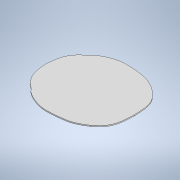
# Autodesk Inventor part: head_1
Saved by Autodesk Inventor 2020 (Build 240168000, 168)
## iProperties
Created: 2022-02-10
Part Number: head_1
Material: Типовые
Document SubType Name: Modeling
Designer: HP
Density: 1 g/cm^3
Appearance: По умолчанию
Mass: 318.083 g
Surface Area: 1630.63 cm^2
Volume: 318.083 cm^3
Author: HP
Autodesk Inventor part; units mm, degrees
ref_plane "YZ Plane" through (0, 0, 0) normal (1, 0, 0) x (0, 1, 0)
ref_plane "XZ Plane" through (0, 0, 0) normal (0, 1, 0) x (-1, 0, 0)
ref_plane "XY Plane" through (0, 0, 0) normal (0, 0, 1) x (1, 0, 0)
sketch "Эскиз1" plane through (0, 0, 0) normal (0, 1, 0) x (-1, 0, 0)
  line L0 (-328.2756, -25.9261) -> (-328.9804, -14.346) construction
  line L1 (-328.9804, -14.346) -> (-329.4417, 0) construction
  line L2 (-329.4417, 0) -> (-328.3635, 17.7121) construction
  line L3 (-328.3635, 17.7121) -> (-327.4394, 35.1161) construction
  line L4 (-327.4394, 35.1161) -> (-325.96, 47.5638) construction
  line L5 (-325.96, 47.5638) -> (-322.3039, 60.9695) construction
  line L6 (-322.3039, 60.9695) -> (-319.1353, 70.8815) construction
  line L7 (-319.1353, 70.8815) -> (-314.3418, 80.4686) construction
  line L8 (-314.3418, 80.4686) -> (-309.3045, 87.4558) construction
  line L9 (-309.3045, 87.4558) -> (-302.3173, 94.9305) construction
  line L10 (-302.3173, 94.9305) -> (-295.98, 101.1053) construction
  line L11 (-295.98, 101.1053) -> (-288.7491, 107.7675) construction
  line L12 (-288.7491, 107.7675) -> (-281.5994, 114.2672) construction
  spline S0 degree 4 poles (-328.2756, -25.9261) (-328.9804, -14.346) (-329.4417, 0) (-328.3635, 17.7121) (-327.4394, 35.1161) (-325.96, 47.5638) (-322.3039, 60.9695) (-319.1353, 70.8815) (-314.3418, 80.4686) (-309.3045, 87.4558) (-302.3173, 94.9305) (-295.98, 101.1053) (-288.7491, 107.7675) (-281.5994, 114.2672) knots 1 1 1 1 1 2 3 4 5 6 7 8 9 10 11 11 11 11 11
  line L13 (-281.5994, 114.2672) -> (-273.0291, 120.561) construction
  line L14 (-273.0291, 120.561) -> (-264.5363, 125.5696) construction
  line L15 (-264.5363, 125.5696) -> (-254.3013, 130.7234) construction
  line L16 (-254.3013, 130.7234) -> (-246.2439, 134.7158) construction
  line L17 (-246.2439, 134.7158) -> (-236.5897, 138.3452) construction
  line L18 (-236.5897, 138.3452) -> (-226.8628, 141.2487) construction
  line L19 (-226.8628, 141.2487) -> (-219.3136, 142.7005) construction
  line L20 (-219.3136, 142.7005) -> (-211.474, 143.9345) construction
  line L21 (-211.474, 143.9345) -> (-203.9248, 144.8781) construction
  line L22 (-203.9248, 144.8781) -> (-196.2304, 145.8944) construction
  line L23 (-196.2304, 145.8944) -> (-187.0117, 147.1284) construction
  line L24 (-187.0117, 147.1284) -> (-177.2848, 147.8543) construction
  line L25 (-177.2848, 147.8543) -> (-168.6468, 148.5076) construction
  line L26 (-168.6468, 148.5076) -> (-161.0976, 148.5076) construction
  line L27 (-161.0976, 148.5076) -> (-152.9677, 149.1609) construction
  line L28 (-152.9677, 149.1609) -> (-144.6926, 149.1609) construction
  line L29 (-144.6926, 149.1609) -> (-134.6028, 147.7817) construction
  spline S1 degree 4 poles (-281.5994, 114.2672) (-273.0291, 120.561) (-264.5363, 125.5696) (-254.3013, 130.7234) (-246.2439, 134.7158) (-236.5897, 138.3452) (-226.8628, 141.2487) (-219.3136, 142.7005) (-211.474, 143.9345) (-203.9248, 144.8781) (-196.2304, 145.8944) (-187.0117, 147.1284) (-177.2848, 147.8543) (-168.6468, 148.5076) (-161.0976, 148.5076) (-152.9677, 149.1609) (-144.6926, 149.1609) (-134.6028, 147.7817) knots 1 1 1 1 1 2 3 4 5 6 7 8 9 10 11 12 13 14 15 15 15 15 15
  line L30 (-134.6028, 147.7817) -> (-125.6357, 146.6668) construction
  line L31 (-125.6357, 146.6668) -> (-119.0855, 145.1103) construction
  line L32 (-119.0855, 145.1103) -> (-109.2278, 141.9974) construction
  line L33 (-109.2278, 141.9974) -> (-99.435, 138.7547) construction
  line L34 (-99.435, 138.7547) -> (-89.1882, 134.4744) construction
  line L35 (-89.1882, 134.4744) -> (-78.4874, 128.8322) construction
  line L36 (-78.4874, 128.8322) -> (-69.2134, 123.3845) construction
  line L37 (-69.2134, 123.3845) -> (-60.588, 117.6774) construction
  line L38 (-60.588, 117.6774) -> (-51.9211, 106.5265) construction
  spline S2 degree 4 poles (-134.6028, 147.7817) (-125.6357, 146.6668) (-119.0855, 145.1103) (-109.2278, 141.9974) (-99.435, 138.7547) (-89.1882, 134.4744) (-78.4874, 128.8322) (-69.2134, 123.3845) (-60.588, 117.6774) (-51.9211, 106.5265) knots 1 1 1 1 1 2 3 4 5 6 7 7 7 7 7
  line L39 (-51.9211, 106.5265) -> (-45.8249, 101.9867) construction
  line L40 (-45.8249, 101.9867) -> (-39.145, 96.9282) construction
  line L41 (-39.145, 96.9282) -> (-31.8815, 90.832) construction
  line L42 (-31.8815, 90.832) -> (-26.1744, 84.1521) construction
  line L43 (-26.1744, 84.1521) -> (-19.9485, 75.2673) construction
  line L44 (-19.9485, 75.2673) -> (-13.8523, 65.669) construction
  line L45 (-13.8523, 65.669) -> (-12.0364, 62.3615) construction
  line L46 (-12.0364, 62.3615) -> (-9.5072, 56.0707) construction
  line L47 (-9.5072, 56.0707) -> (-5.8754, 44.462) construction
  line L48 (-5.8754, 44.462) -> (-2.957, 29.6755) construction
  line L49 (-2.957, 29.6755) -> (-1.0763, 17.7425) construction
  line L50 (-1.0763, 17.7425) -> (0.1559, 5.3556) construction
  line L51 (0.1559, 5.3556) -> (0.1559, -6.1883) construction
  line L52 (0.1559, -6.1883) -> (-0.8168, -22.8555) construction
  line L53 (-0.8168, -22.8555) -> (-2.3085, -36.4747) construction
  spline S3 degree 4 poles (-51.9211, 106.5265) (-45.8249, 101.9867) (-39.145, 96.9282) (-31.8815, 90.832) (-26.1744, 84.1521) (-19.9485, 75.2673) (-13.8523, 65.669) (-12.0364, 62.3615) (-9.5072, 56.0707) (-5.8754, 44.462) (-2.957, 29.6755) (-1.0763, 17.7425) (0.1559, 5.3556) (0.1559, -6.1883) (-0.8168, -22.8555) (-2.3085, -36.4747) knots 1 1 1 1 1 2 3 4 5 6 7 8 9 10 11 12 13 13 13 13 13
  line L54 (-329.4417, 0) -> (0, 0)
  line L55 (-328.2756, 25.9261) -> (-328.9804, 14.346) construction
  line L56 (-328.9804, 14.346) -> (-329.4417, 0) construction
  line L57 (-329.4417, 0) -> (-328.3635, -17.7121) construction
  line L58 (-328.3635, -17.7121) -> (-327.4394, -35.1161) construction
  line L59 (-327.4394, -35.1161) -> (-325.96, -47.5638) construction
  line L60 (-325.96, -47.5638) -> (-322.3039, -60.9695) construction
  line L61 (-322.3039, -60.9695) -> (-319.1353, -70.8815) construction
  line L62 (-319.1353, -70.8815) -> (-314.3418, -80.4686) construction
  line L63 (-314.3418, -80.4686) -> (-309.3045, -87.4558) construction
  line L64 (-309.3045, -87.4558) -> (-302.3173, -94.9305) construction
  line L65 (-302.3173, -94.9305) -> (-295.98, -101.1053) construction
  line L66 (-295.98, -101.1053) -> (-288.7491, -107.7675) construction
  line L67 (-288.7491, -107.7675) -> (-281.5994, -114.2672) construction
  spline S4 degree 4 poles (-328.2756, 25.9261) (-328.9804, 14.346) (-329.4417, 0) (-328.3635, -17.7121) (-327.4394, -35.1161) (-325.96, -47.5638) (-322.3039, -60.9695) (-319.1353, -70.8815) (-314.3418, -80.4686) (-309.3045, -87.4558) (-302.3173, -94.9305) (-295.98, -101.1053) (-288.7491, -107.7675) (-281.5994, -114.2672) knots 1 1 1 1 1 2 3 4 5 6 7 8 9 10 11 11 11 11 11
  line L68 (-281.5994, -114.2672) -> (-273.0291, -120.561) construction
  line L69 (-273.0291, -120.561) -> (-264.5363, -125.5696) construction
  line L70 (-264.5363, -125.5696) -> (-254.3013, -130.7234) construction
  line L71 (-254.3013, -130.7234) -> (-246.2439, -134.7158) construction
  line L72 (-246.2439, -134.7158) -> (-236.5897, -138.3452) construction
  line L73 (-236.5897, -138.3452) -> (-226.8628, -141.2487) construction
  line L74 (-226.8628, -141.2487) -> (-219.3136, -142.7005) construction
  line L75 (-219.3136, -142.7005) -> (-211.474, -143.9345) construction
  line L76 (-211.474, -143.9345) -> (-203.9248, -144.8781) construction
  line L77 (-203.9248, -144.8781) -> (-196.2304, -145.8944) construction
  line L78 (-196.2304, -145.8944) -> (-187.0117, -147.1284) construction
  line L79 (-187.0117, -147.1284) -> (-177.2848, -147.8543) construction
  line L80 (-177.2848, -147.8543) -> (-168.6468, -148.5076) construction
  line L81 (-168.6468, -148.5076) -> (-161.1015, -148.2639) construction
  line L82 (-161.1015, -148.2639) -> (-152.9547, -148.6545) construction
  line L83 (-152.9547, -148.6545) -> (-144.6926, -149.1609) construction
  line L84 (-144.6926, -149.1609) -> (-134.6028, -147.7817) construction
  spline S5 degree 4 poles (-281.5994, -114.2672) (-273.0291, -120.561) (-264.5363, -125.5696) (-254.3013, -130.7234) (-246.2439, -134.7158) (-236.5897, -138.3452) (-226.8628, -141.2487) (-219.3136, -142.7005) (-211.474, -143.9345) (-203.9248, -144.8781) (-196.2304, -145.8944) (-187.0117, -147.1284) (-177.2848, -147.8543) (-168.6468, -148.5076) (-161.1015, -148.2639) (-152.9547, -148.6545) (-144.6926, -149.1609) (-134.6028, -147.7817) knots 1 1 1 1 1 2 3 4 5 6 7 8 9 10 11 12 13 14 15 15 15 15 15
  line L85 (-134.6028, -147.7817) -> (-125.6357, -146.6668) construction
  line L86 (-125.6357, -146.6668) -> (-119.0855, -145.1103) construction
  line L87 (-119.0855, -145.1103) -> (-109.3334, -141.6808) construction
  line L88 (-109.3334, -141.6808) -> (-99.435, -138.7547) construction
  line L89 (-99.435, -138.7547) -> (-89.1882, -134.4744) construction
  line L90 (-89.1882, -134.4744) -> (-78.4874, -128.8322) construction
  line L91 (-78.4874, -128.8322) -> (-69.2134, -123.3845) construction
  line L92 (-69.2134, -123.3845) -> (-60.588, -117.6774) construction
  line L93 (-60.588, -117.6774) -> (-51.9211, -106.5265) construction
  spline S6 degree 4 poles (-134.6028, -147.7817) (-125.6357, -146.6668) (-119.0855, -145.1103) (-109.3334, -141.6808) (-99.435, -138.7547) (-89.1882, -134.4744) (-78.4874, -128.8322) (-69.2134, -123.3845) (-60.588, -117.6774) (-51.9211, -106.5265) knots 1 1 1 1 1 2 3 4 5 6 7 7 7 7 7
  line L94 (-51.9211, -106.5265) -> (-45.8249, -101.9867) construction
  line L95 (-45.8249, -101.9867) -> (-39.145, -96.9282) construction
  line L96 (-39.145, -96.9282) -> (-31.8815, -90.832) construction
  line L97 (-31.8815, -90.832) -> (-26.1744, -84.1521) construction
  line L98 (-26.1744, -84.1521) -> (-19.9485, -75.2673) construction
  line L99 (-19.9485, -75.2673) -> (-13.8523, -65.669) construction
  line L100 (-13.8523, -65.669) -> (-12.0364, -62.3615) construction
  line L101 (-12.0364, -62.3615) -> (-9.5072, -56.0707) construction
  line L102 (-9.5072, -56.0707) -> (-5.8754, -44.462) construction
  line L103 (-5.8754, -44.462) -> (-2.957, -29.6755) construction
  line L104 (-2.957, -29.6755) -> (-1.0763, -17.7425) construction
  line L105 (-1.0763, -17.7425) -> (0.1559, -5.3556) construction
  line L106 (0.1559, -5.3556) -> (0.1559, 6.1883) construction
  line L107 (0.1559, 6.1883) -> (-0.8168, 22.8555) construction
  line L108 (-0.8168, 22.8555) -> (-2.3085, 36.4747) construction
  spline S7 degree 4 poles (-51.9211, -106.5265) (-45.8249, -101.9867) (-39.145, -96.9282) (-31.8815, -90.832) (-26.1744, -84.1521) (-19.9485, -75.2673) (-13.8523, -65.669) (-12.0364, -62.3615) (-9.5072, -56.0707) (-5.8754, -44.462) (-2.957, -29.6755) (-1.0763, -17.7425) (0.1559, -5.3556) (0.1559, 6.1883) (-0.8168, 22.8555) (-2.3085, 36.4747) knots 1 1 1 1 1 2 3 4 5 6 7 8 9 10 11 12 13 13 13 13 13
  point P0 (0, 0)
  point P1 (-0.5497, -16.6468)
  point P2 (0, 0)
  point P3 (-1.0867, 16.6204)
  point P4 (-329.0787, 0)
  dimension "d29" = 295.5634
  constraints: 51 symmetric about line, 3 horizontal, 2 end point, 1 coincident, 1 vertical, 25 other
  measures "d29" distance of L29.end L84.end
extrude "Выдавливание1" add sketch "Эскиз1" along normal blind 4
